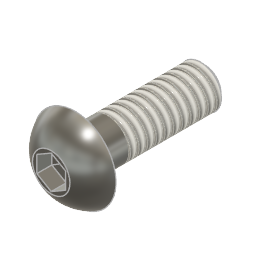
grognatiny (Autodesk Fusion 360 archive; units mm, degrees)
design "Hexagon Socket Button Head Screw ISO 7380-1 - M2 x 6 Steel 4.6 Plain"
description: Hexagon Socket Button Head Screw ISO 7380-1 - M2 x 6
part number: ISO 7380-1 - M2 x 6 Steel 4.6 Plain
Autodesk Fusion 360 part; units mm, degrees
sketch "Sketch1" plane through (0, 0, 0) normal (0, 1, 0) x (1, 0, 0)
  line L0 (-1, 0) -> (-1, 6)
  line L1 (-1, 6) -> (0, 6)
  line L2 (0, 6) -> (0, -1.1)
  line L3 (-1, 0) -> (-1.9, 0)
  line L4 (0, -1.1) -> (-0.8667, -1.1)
  arc A0 (-1.9, 0) -> (-0.8667, -1.1) centre (0, 0.7495) ccw
  dimension "d9" = 2
  dimension "d66" = 3.8
  dimension "d98" = 1.7333
  dimension "d105" = 1.1
  dimension "d106" = 6
  constraint perpendicular L0 L1
  constraint perpendicular L0 L3
  constraint coincident origin L3
  constraint vertical L0
  constraint vertical L2
  constraint coincident origin L2
  constraint perpendicular L2 L4
  constraint coincident L2 A0.centre
  measures "d105" distance of L3 L4
  measures "d106" distance of origin L1
revolve "Revolve1" add sketch "Sketch1" angle 360 about axis through (0, 0, -6) along (0, 0, 1)
ref_plane "WorkPlane1" through (0, 0, 1.1) normal (0, 0, 1) x (1, 0, 0)
sketch "Sketch6" plane through (0, 0, 1.1) normal (0, 0, 1) x (1, 0, 0)
  line L0 (0, -0.7698) -> (0.6667, -0.3849)
  line L1 (0.6667, -0.3849) -> (0.6667, 0.3849)
  line L2 (0.6667, 0.3849) -> (0, 0.7698)
  line L3 (0, 0.7698) -> (-0.6667, 0.3849)
  line L4 (-0.6667, 0.3849) -> (-0.6667, -0.3849)
  line L5 (-0.6667, -0.3849) -> (0, -0.7698)
  dimension "d117" = 1.3333
  constraint vertical L1
  measures "d117" distance of L1 L4
extrude "Extrude1" cut sketch "Sketch6" against normal blind 0.6933
extrude "Extrude2" cut 1 faces at (-0.2222, 0.1283, 0.4067) along direction (0, 0, -1) blind 0.6933 draft -85
fillet "Fillet5" radius 0.2 1 edges at (-0.9323, 0.3616, 0)
thread "Thread5" "ISO Metric profile 2.0 M2x0.4 M2x0.4 6g" major diameter 1.9335 minor diameter 1.478 pitch 0.4 angle 60 resizes the face on face at (-0.9988, 0.0498, -2.1333) from (0, 0, -1.5) to (0, 0, -6)
sketch "Sketch5" plane through (0, 0, 0) normal (0, 1, 0) x (1, 0, 0)
  line L0 (0, 6) -> (0, -1.1)
  line L1 (0, 6) -> (-1.02, 6)
  line L2 (-1.02, 6) -> (-1.02, 5.7546)
  line L3 (-1.02, 5.7546) -> (-0.7546, 6)
  dimension "d108" = 0.2454
  dimension "d109" = 0.7546
  dimension "d110" = 1.02
  constraint coincident L0.start L1.start
  constraint perpendicular L1 L2
  constraint coincident L1 L3.end
  measures "d108" distance of L1 L2.end
  measures "d109" distance of L0 L3.end
  measures "d110" distance of L0 L2
revolve "Revolve2" cut sketch "Sketch5" angle 360 about axis through (0, 0, -6) along (0, 0, 1)
equation "d9 = adsk_nomdia"
equation "adsk_nomlen = 6.00 mm"
equation "adsk_headh = 1.10 mm"
equation "adsk_headdia = 3.80 mm"
equation "adsk_nomdia = 2.00 mm"
equation "adsk_philwidth = 1.3333333 mm"
equation "d31 = -adsk_phildepth"
equation "adsk_phildepth = 0.6933333 mm"
equation "d66 = adsk_headdia"
equation "d71 = adsk_headh"
equation "d76 = -adsk_phildepth"
equation "adsk_thrlen = 4.50 mm"
equation "adsk_endpointdia = 1.50924 mm"
equation "adsk_startlen = 0.24538 mm"
equation "d98 = adsk_philwidth * 1.3"
equation "adsk_midfillet = 0.20 mm"
equation "d104 = adsk_midfillet"
equation "d105 = adsk_headh"
equation "d106 = adsk_nomlen"
equation "d108 = adsk_startlen"
equation "d109 = adsk_endpointdia / 2"
equation "d110 = adsk_nomdia * 0.51"
equation "d116 = min(adsk_thrlen; adsk_nomlen - adsk_midfillet - 0.001 mm)"
equation "d117 = adsk_philwidth"
